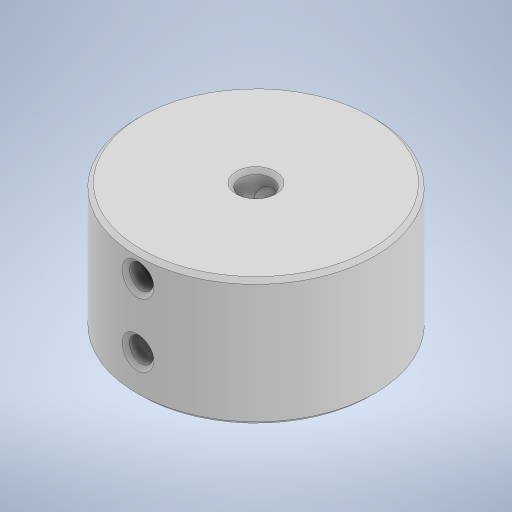
# Autodesk Inventor part: Втулка энкодера штурвала
Saved by Autodesk Inventor 2023 (Build 270158000, 158)
## iProperties
Created: 2022-05-17
Part Number: Втулка энкодера штурвала
Material: Типовые
Document SubType Name: Modeling
Designer: avkap
Density: 1 g/cm^3
Appearance: По умолчанию
Author: avkap
Autodesk Inventor part; units mm, degrees
ref_plane "YZ Plane" through (0, 0, 0) normal (1, 0, 0) x (0, 1, 0)
ref_plane "XZ Plane" through (0, 0, 0) normal (0, 1, 0) x (-1, 0, 0)
ref_plane "XY Plane" through (0, 0, 0) normal (0, 0, 1) x (1, 0, 0)
sketch "Эскиз1" plane through (0, 0, 0) normal (0, 1, 0) x (-1, 0, 0)
  circle A0 centre (0, 0) radius 12.5
  circle A1 centre (0, 0) radius 15
  dimension "d0" = 25
  dimension "d1" = 30
  constraints: 2 centre point, 2 coincident
  measures "d0" diameter of A0
  measures "d1" diameter of A1
extrude "Выдавливание1" add sketch "Эскиз1" along normal blind 10
sketch "Эскиз2" plane through (0, 10, 0) normal (0, 1, 0) x (1, 0, 0)
  circle A0 centre (0, 0) radius 15
  circle A1 centre (0, 0) radius 2
  dimension "d4" = 4
  constraints: 2 centre point, 2 coincident
  measures "d4" diameter of A1
extrude "Выдавливание2" add sketch "Эскиз2" along normal blind 6
sketch "Эскиз3" plane through (0, 0, 0) normal (0, 0, 1) x (1, 0, 0)
  line L0 (0, 0) -> (0, 5)
  line L1 (15, 16) -> (-15, 16) projected
  line L2 (0, 16) -> (0, 13)
  circle A0 centre (0, 13) radius 1.5
  circle A1 centre (0, 5) radius 1.5
  dimension "d7" = 5
  dimension "d8" = 3
  dimension "d9" = 3
  dimension "d10" = 3
  constraints: 4 end point, 2 centre point, 2 coincident, 1 midpoint, 1 point on line, 1 vertical
  measures "d7" distance of L0.start L0.end
  measures "d8" distance of L2.start L2.end
  measures "d9" diameter of A0
  measures "d10" diameter of A1
extrude "Выдавливание3" cut sketch "Эскиз3" along normal blind 29 and the other way blind 25.5
chamfer "Фаска1" distance 0.5 angle 45 8 edges at (-1.5, 12.998, 14.9248) (-1.5, 4.998, 14.9248) (-2, 16, 0) (-1.5, 12.998, -14.9248) (-1.5, 4.998, -14.9248) (12.5, 0, 0) (15, 0, 0) (-15, 16, 0)
